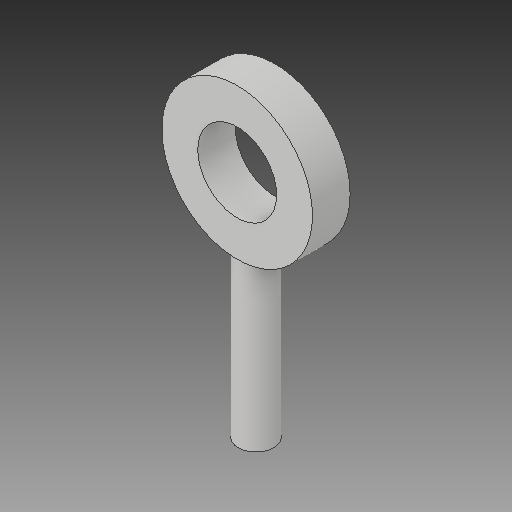
# Autodesk Inventor part: eye screw stand-in
Saved by Autodesk Inventor 2018 (Build 220112000, 112)
## iProperties
Created: 2019-03-01
Part Number: eye screw stand-in
Material: Generic
Document SubType Name: Modeling
Designer: s-2513225
Density: 1 g/cm^3
Appearance: Default
Author: s-2513225
Autodesk Inventor part; units mm, degrees
ref_plane "XY Plane" through (0, 0, 0) normal (0, 0, 1) x (1, 0, 0)
ref_plane "Work Plane1" through (6.5151, 0, 0) normal (1, 0, 0) x (0, 1, 0)
sketch "Sketch2" plane through (0, 0, 0) normal (0, 0, 1) x (1, 0, 0)
  circle A0 centre (0, 0) radius 8.636
  circle A1 centre (0, 0) radius 4.5212
  line L0 (0, -8.636) -> (0, -27.432) construction
  dimension "d2" = 17.272
  dimension "d3" = 4.1148
  dimension "d4" = 18.796
  constraints: 2 end point, 1 centre point, 1 coincident, 1 vertical, 1 vertical alignment, 2 other
  measures "d4" distance of L0.start L0.end
extrude "Extrusion1" add sketch "Sketch2" along normal mid plane 4.318
ref_plane "Work Plane2" through (0, -8.6106, 0) normal (0, 1, 0) x (-1, 0, 0)
sketch "Sketch3" plane through (0, -8.6106, 0) normal (0, 1, 0) x (-1, 0, 0)
  circle A0 centre (0, 0) radius 2.0574
  dimension "d8" = 4.1148
  constraints: 1 centre point, 1 coincident
  measures "d8" diameter of A0
extrude "Extrusion2" add sketch "Sketch3" against normal blind 18.796
body "Solid1"
